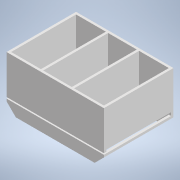
# Autodesk Inventor part: BeadCompartments_5
Saved by Autodesk Inventor 2020 (Build 240168000, 168)
## iProperties
Created: 2022-01-22
Part Number: BeadCompartments_5
Material: Generic
Document SubType Name: Modeling
Designer: danie
Density: 1 g/cm^3
Appearance: Default
Author: danie
Autodesk Inventor part; units mm, degrees
ref_plane "YZ Plane" through (0, 0, 0) normal (1, 0, 0) x (0, 1, 0)
ref_plane "XZ Plane" through (0, 0, 0) normal (0, 1, 0) x (-1, 0, 0)
ref_plane "XY Plane" through (0, 0, 0) normal (0, 0, 1) x (1, 0, 0)
sketch "Sketch1" plane through (0, 0, 0) normal (0, 1, 0) x (-1, 0, 0)
  line L0 (0, 0) -> (0, -88.9)
  line L1 (0, -88.9) -> (-127, -88.9)
  line L2 (-127, -88.9) -> (-127, 0)
  line L3 (-127, 0) -> (0, 0)
  line L4 (3.175, -92.075) -> (3.175, 3.175)
  line L5 (3.175, 3.175) -> (-130.175, 3.175)
  line L6 (-130.175, 3.175) -> (-130.175, -92.075)
  line L7 (-130.175, -92.075) -> (3.175, -92.075)
  line L8 (0, 0) -> (0, -88.9)
  line L9 (0, -88.9) -> (-40.7416, -88.9)
  line L10 (-40.7416, -88.9) -> (-40.7416, 0)
  line L11 (-40.7416, 0) -> (0, 0)
  line L12 (-40.7416, 0) -> (-40.7416, -88.9)
  line L13 (-40.7416, -88.9) -> (-43.9166, -88.9)
  line L14 (-43.9166, -88.9) -> (-43.9166, 0)
  line L15 (-43.9166, 0) -> (-40.7416, 0)
  line L16 (-127, -88.9) -> (-127, 0)
  line L17 (-127, 0) -> (-86.2584, 0)
  line L18 (-86.2584, 0) -> (-86.2584, -88.9)
  line L19 (-86.2584, -88.9) -> (-127, -88.9)
  line L20 (-86.2584, 0) -> (-86.2584, -88.9)
  line L21 (-86.2584, -88.9) -> (-83.0834, -88.9)
  line L22 (-83.0834, -88.9) -> (-83.0834, 0)
  line L23 (-83.0834, 0) -> (-86.2584, 0)
  dimension "d0" = 88.9
  dimension "d1" = 127
  dimension "d2" = 3.175
  dimension "d3" = 40.7416
  dimension "d4" = 3.175
  dimension "d5" = 40.7416
  dimension "d6" = 3.175
  constraints: 48 end point, 13 parallel, 7 perpendicular, 2 collinear, 1 vertical, 3 other
  measures "d0" distance of L0.start L0.end
  measures "d1" distance of L0.end L1.end
  measures "d2" distance between parallel lines of L0 L4
  measures "d3" distance of L0.end L9.end
  measures "d4" distance of L9.end L13.end
  measures "d5" distance of L2.end L17.end
  measures "d6" distance of L21.end L18.end
extrude "Extrusion1" add sketch "Sketch1" along normal blind 50.8 contours L10 L1 L14 L3 | L22 L1 L18 L3 | L7 L6 L5 L4
sketch "Sketch2" plane through (0, 0, 0) normal (0, -1, 0) x (1, 0, 0)
  line L0 (-3.175, 3.175) -> (130.175, 3.175) projected
  line L1 (-3.175, 3.175) -> (130.175, 3.175)
  line L2 (130.175, 3.175) -> (130.175, 0)
  line L3 (130.175, 0) -> (-3.175, 0)
  line L4 (-3.175, 0) -> (-3.175, 3.175)
  point P0 (0, 0)
  constraints: 8 end point, 3 equal length, 1 perpendicular
extrude "Extrusion2" add sketch "Sketch2" along normal blind 2.54
sketch "Sketch3" plane through (0, 0, 0) normal (0, -1, 0) x (1, 0, 0)
  line L0 (130.175, -92.075) -> (-3.175, -92.075) projected
  line L1 (-3.175, -92.075) -> (130.175, -92.075)
  line L2 (130.175, -92.075) -> (130.175, -88.9)
  line L3 (130.175, -88.9) -> (-3.175, -88.9)
  line L4 (-3.175, -88.9) -> (-3.175, -92.075)
  point P0 (0, 0)
  dimension "d11" = 3.175
  constraints: 8 end point, 2 parallel, 1 horizontal, 1 perpendicular
  measures "d11" distance of L2.end L0.start
extrude "Extrusion3" add sketch "Sketch3" along normal blind 7.62
sketch "Sketch4" plane through (0, -7.62, 0) normal (0, -1, 0) x (1, 0, 0)
  line L0 (130.175, -92.075) -> (-3.175, -92.075) projected
  line L1 (-3.175, -92.075) -> (130.175, -92.075)
  line L2 (130.175, -92.075) -> (130.175, 3.175)
  line L3 (130.175, 3.175) -> (-3.175, 3.175)
  line L4 (-3.175, 3.175) -> (-3.175, -92.075)
  line L5 (0, 0) -> (127, 0)
  line L6 (127, 0) -> (127, -88.9)
  line L7 (127, -88.9) -> (0, -88.9)
  line L8 (0, -88.9) -> (0, 0)
  point P0 (0, 0)
  constraints: 16 end point, 4 parallel, 2 perpendicular, 1 horizontal, 3 other
extrude "Extrusion4" add sketch "Sketch4" against normal blind 3.175
sketch "Sketch9" plane through (-3.175, -7.62, 3.175) normal (0, 0, 1) x (1, 0, 0)
  line L0 (0, 58.42) -> (0, 0) construction
  line L1 (0, 0) -> (0, -12.7) construction
  line L2 (0, -12.7) -> (0, 0) construction
  line L3 (0, -12.7) -> (12.7, -12.7) construction
  line L4 (0, 0) -> (133.35, 0) construction
  line L5 (133.35, 0) -> (133.35, -12.7) construction
  line L6 (133.35, -12.7) -> (120.65, -12.7) construction
  line L7 (0, 0) -> (12.7, -12.7)
  line L8 (12.7, -12.7) -> (120.65, -12.7)
  line L9 (120.65, -12.7) -> (133.35, 0)
  line L10 (0, 0) -> (133.35, 0)
  point P0 (3.175, 7.62)
  dimension "d28" = 12.7
  dimension "d29" = 12.7
  dimension "d30" = 90
  dimension "d31" = 12.7
  dimension "d32" = 12.7
  constraints: 18 end point, 3 vertical, 2 perpendicular, 1 collinear, 1 horizontal
  measures "d28" distance of L0.end L1.end
  measures "d29" distance of L1.end L0.end
  measures "d30" angle of L3 L2
  measures "d31" distance of L4.end L5.end
  measures "d32" distance of L5.end L6.end
extrude "Extrusion9" add sketch "Sketch9" against normal blind 3.175
sketch "Sketch10" plane through (130.175, 50.8, -92.075) normal (0, 0, -1) x (-1, 0, 0)
  line L0 (133.35, -58.42) -> (0, -58.42) projected
  line L1 (12.7, -71.12) -> (120.65, -71.12) projected
  line L2 (133.35, -58.42) -> (120.65, -71.12)
  line L3 (0, -58.42) -> (12.7, -71.12) projected
  line L4 (120.65, -71.12) -> (12.7, -71.12)
  line L5 (12.7, -71.12) -> (0, -58.42)
  line L6 (0, -58.42) -> (133.35, -58.42)
  point P0 (130.175, -50.8)
  constraints: 8 end point, 1 collinear, 1 horizontal, 1 parallel
extrude "Extrusion10" add sketch "Sketch10" against normal blind 3.175
sketch "Sketch11" plane through (130.175, -7.62, -88.9) normal (0.7071068, -0.7071068, 0) x (-0.7071068, -0.7071068, 0)
  line L0 (0, 3.175) -> (0, 0) projected
  line L1 (17.9605, 3.175) -> (17.9605, 0) projected
  line L2 (0, 3.175) -> (17.9605, 3.175)
  line L3 (17.9605, 3.175) -> (17.9605, -92.075)
  line L4 (17.9605, -92.075) -> (0, -92.075)
  line L5 (0, -92.075) -> (0, 3.175)
  point P0 (86.6595, -88.9)
  constraints: 8 end point, 2 parallel, 1 horizontal, 1 perpendicular
extrude "Extrusion11" add sketch "Sketch11" against normal blind 3.175
sketch "Sketch12" plane through (9.525, -20.32, -88.9) normal (-0.7071068, -0.7071068, 0) x (-0.7071068, 0.7071068, 0)
  line L0 (59.2697, 3.175) -> (17.9605, 3.175) projected
  line L1 (17.9605, -92.075) -> (0, -92.075) projected
  line L2 (17.9605, 3.175) -> (17.9605, -92.075)
  line L3 (17.9605, -92.075) -> (0, -92.075)
  line L4 (0, -92.075) -> (0, 3.175)
  line L5 (0, 3.175) -> (17.9605, 3.175)
  point P0 (21.1036, -88.9)
  point P1 (0, -92.075)
  constraints: 8 end point, 2 parallel, 1 perpendicular, 1 vertical
extrude "Extrusion12" add sketch "Sketch12" against normal blind 3.175
sketch "Sketch13" plane through (127, 0, -88.9) normal (-1, 0, 0) x (0, 0, 1)
  line L0 (0, 50.8) -> (9.525, 50.8) construction
  line L1 (0, 50.8) -> (88.9, 50.8) construction
  line L2 (9.525, 50.8) -> (9.525, 44.45) construction
  circle A0 centre (9.525, 44.45) radius 2.3876
  line L3 (9.525, 44.45) -> (73.025, 44.45) construction
  circle A1 centre (73.025, 44.45) radius 2.3876
  point P0 (88.9, 0)
  dimension "d46" = 9.525
  dimension "d47" = 6.35
  dimension "d48" = 4.7752
  dimension "d49" = 63.5
  dimension "d50" = 4.7752
  constraints: 6 end point, 2 centre point, 2 coincident, 1 horizontal, 1 perpendicular, 1 point on line
  measures "d46" distance of L0.start L0.end
  measures "d47" distance of L0.end L2.end
  measures "d48" diameter of A0
  measures "d49" distance of L3.start L3.end
  measures "d50" diameter of A1
extrude "Extrusion13" cut sketch "Sketch13" against normal blind 3.175
sketch "Sketch14" plane through (130.175, 50.8, -92.075) normal (0, 0, -1) x (-1, 0, 0)
  line L0 (0, -53.34) -> (0, 0) construction
  line L1 (0, 0) -> (0, -6.35) construction
  line L2 (0, -6.35) -> (9.5244, -6.2428) construction
  line L3 (9.5244, -6.2428) -> (98.4244, -6.2428) construction
  circle A0 centre (9.5244, -6.2428) radius 2.3876
  circle A1 centre (98.4244, -6.2428) radius 2.3876
  point P0 (130.175, -50.8)
  dimension "d51" = 6.35
  dimension "d52" = 9.525
  dimension "d53" = 88.9
  dimension "d54" = 4.7752
  dimension "d55" = 4.7752
  constraints: 6 end point, 2 centre point, 2 coincident, 1 horizontal, 1 point on line
  measures "d51" distance of L0.end L1.end
  measures "d52" distance of L1.end L2.end
  measures "d53" distance of L2.end L3.end
  measures "d54" diameter of A0
  measures "d55" diameter of A1
extrude "Extrusion14" cut sketch "Sketch14" against normal blind 3.175
body "Solid1"
